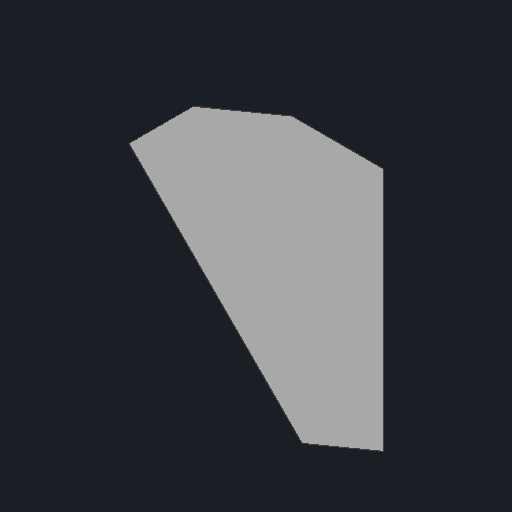
# Autodesk Inventor part: DMF 01 57 Сетка кассеты v2.1
Saved by Autodesk Inventor 2026.2 (Build 302298000, 298)
## iProperties
Created: 2024-05-05
Part Number: DMF 01 57 Сетка кассеты v2.1
Material: Generic
Document SubType Name: Modeling
Designer: pokla
Density: 1 g/cm^3
Appearance: Default
Sheet Metal Rule: Default
Author: pokla
Autodesk Inventor part; units mm, degrees
ref_plane "YZ Plane" through (0, 0, 0) normal (1, 0, 0) x (0, 1, 0)
ref_plane "XZ Plane" through (0, 0, 0) normal (0, 1, 0) x (-1, 0, 0)
ref_plane "XY Plane" through (0, 0, 0) normal (0, 0, 1) x (1, 0, 0)
sketch "Sketch1" plane through (0, 0, 0) normal (0, 0, 1) x (1, 0, 0)
  line L0 (0, 278.716) -> (197.082, 197.082) construction
  line L1 (197.082, 197.082) -> (278.716, 0) construction
  line L2 (278.716, 0) -> (197.082, -197.082) construction
  line L3 (197.082, -197.082) -> (0, -278.716) construction
  line L4 (0, -278.716) -> (-197.082, -197.082) construction
  line L5 (-197.082, -197.082) -> (-278.716, 0) construction
  line L6 (-278.716, 0) -> (-197.082, 197.082) construction
  line L7 (-197.082, 197.082) -> (0, 278.716)
  line L8 (-197.082, 197.082) -> (0, 278.716)
  line L9 (-461.6493, 774.8136) -> (-221.4406, 874.3113)
  line L10 (-98.541, 237.899) -> (-341.545, 824.5625) construction
  line L11 (-221.4406, 874.3113) -> (0, 874.3113)
  line L12 (0, 874.3113) -> (0, 278.716)
  line L13 (-461.6493, 774.8136) -> (-618.2315, 618.2315)
  line L14 (-618.2315, 618.2315) -> (-197.082, 197.082)
  point P0 (0, 0)
  point P1 (0, 0)
  dimension "d0" = 515
  dimension "d2" = 260
  dimension "d3" = 635
  constraints: 30 end point, 2 midpoint, 1 coincident, 1 horizontal, 1 parallel, 1 perpendicular, 1 symmetric about line, 1 vertical, 1 vertical alignment, 17 other
  measures "d0" distance between parallel lines of L5 L1
  measures "d2" distance of L9.start L9.end
  measures "d3" distance of L10.end L10.start
extrude "Extrusion1" add sketch "Sketch1" along normal mid plane 0.5
sketch "Sketch7" plane through (0, 0, 0.25) normal (0, 0, 1) x (1, 0, 0)
  line L0 (-13, 869.3113) -> (-5, 869.3113)
  line L1 (-5, 869.3113) -> (-5, 861.3113)
  line L2 (-5, 861.3113) -> (-13, 861.3113)
  line L3 (-13, 861.3113) -> (-13, 869.3113)
  line L4 (0, 874.3113) -> (-221.4406, 874.3113) projected
  line L5 (0, 278.716) -> (0, 874.3113) projected
  point P0 (0, 0)
  dimension "d54" = 8
  dimension "d55" = 8
  dimension "d56" = 5
  dimension "d57" = 5
  constraints: 8 end point, 2 parallel, 1 horizontal, 1 perpendicular
  measures "d54" distance of L1.end L2.end
  measures "d55" distance of L0.end L1.end
  measures "d56" distance between parallel lines of L4 L0
  measures "d57" distance between parallel lines of L5 L1
extrude "Extrusion5" [suppressed]
pattern_linear "Rectangular Pattern1" [suppressed]
equation "\"d0\" = Барабан_размер_по_плоскостям"
equation "\"d2\" = Кассета_длина_грани"
equation "\"d3\" = Кассета_высота"
equation "\"BendRadius\" = Thickness"
equation "\"BendReliefWidth\" = Thickness"
equation "\"BendReliefDepth\" = 0.5 * Thickness"
equation "\"CornerReliefSize\" = 4 * Thickness"
equation "\"MinimumRemnant\" = 2 * Thickness"
equation "\"TransitionRadius\" = BendRadius"
equation "\"JacobiRadiusSize\" = BendRadius"
equation "\"GapSize\" = Thickness"
equation "\"Барабан_размер_по_плоскостям\" = 515"
equation "\"Кассета_длина_грани\" = 260"
equation "\"Кассета_высота\" = 635"
equation "\"Thickness\" = 0.5"
body "Solid1"
